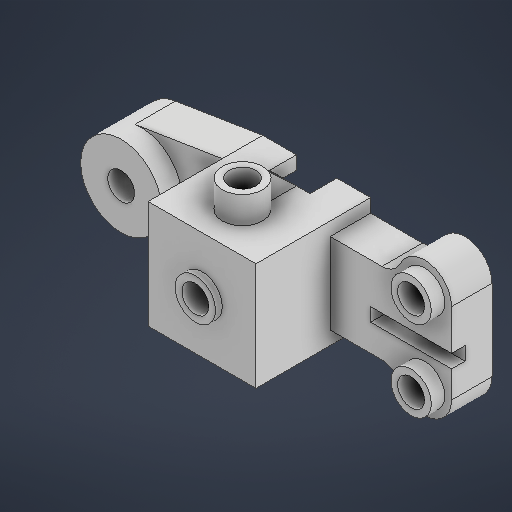
# Autodesk Inventor part: b5
Saved by Autodesk Inventor 2025.4 (Build 294407000, 407)
## iProperties
Created: 2026-05-15
Part Number: b5
Material: Generic
Document SubType Name: Modeling
Designer: VuQuan
Density: 1 g/cm^3
Appearance: Default
Author: VuQuan
Autodesk Inventor part; units mm, degrees
ref_plane "YZ Plane" through (0, 0, 0) normal (1, 0, 0) x (0, 1, 0)
ref_plane "XZ Plane" through (0, 0, 0) normal (0, 1, 0) x (-1, 0, 0)
ref_plane "XY Plane" through (0, 0, 0) normal (0, 0, 1) x (1, 0, 0)
sketch "Sketch1" plane through (0, 0, 0) normal (0, 0, 1) x (1, 0, 0)
  circle A0 centre (0, 0) radius 30
  line L0 (60, 40) -> (140, 40)
  line L1 (140, 40) -> (140, -40)
  line L2 (140, -40) -> (60, -40)
  line L3 (60, -40) -> (60, 40)
  line L4 (60, 40) -> (-4.7479, 29.6219)
  line L5 (60, -40) -> (-4.7479, -29.6219)
  line L6 (140, 30) -> (178.3772, 30)
  arc A1 (230, 30) -> (191.9298, 38.5714) centre (210, 30) ccw
  line L7 (230, 30) -> (230, -30)
  arc A2 (191.9298, -38.5714) -> (230, -30) centre (210, -30) ccw
  line L8 (178.3772, -30) -> (140, -30)
  arc A3 (178.3772, 30) -> (191.9298, 38.5714) centre (178.3772, 45) ccw
  arc A4 (191.9298, -38.5714) -> (178.3772, -30) centre (178.3772, -45) ccw
  point P0 (60, 0)
  point P1 (100, -40)
  point P2 (190, 30)
  point P3 (190, -30)
  point P4 (230, 0)
  point P5 (140, 0)
  dimension "d0" = 60
  dimension "d1" = 80
  dimension "d2" = 100
  dimension "d3" = 60
  dimension "d4" = 20
  dimension "d5" = 110
  dimension "d61" = 15
  constraints: 18 end point, 12 point on circle, 8 tangent, 7 point on line, 5 centre point, 4 midpoint, 4 perpendicular, 2 horizontal, 2 horizontal alignment, 2 parallel, 1 coincident, 1 equal radius, 1 vertical alignment
  measures "d0" diameter of A0
  measures "d1" distance of L1.end L2.end
  measures "d2" horizontal distance of point (100, -40) point (0, 0)
  measures "d3" distance between parallel lines of L8 L6
  measures "d4" radius of A1
  measures "d5" horizontal distance of A2.centre point (100, -40)
  measures "d61" radius of A3
extrude "Extrusion1" add sketch "Sketch1" along normal blind 45 contours A0
extrude "Extrusion2" add sketch "Sketch1" along normal blind 30 contours A0 L4 L3 L5 | L6 A3 A1 L7 A2 A4 L8 L1
extrude "Extrusion3" add sketch "Sketch1" along normal blind 85 contours L0 L1 L2 L3
hole "Hole1" at (0, 0, 0) direction (0, 0, 1) diameter 20 depth 45
sketch "Sketch2" plane through (0, 0, 0) normal (0, 0, -1) x (-1, 0, 0)
  circle A0 centre (0, 0) radius 10 projected
  line L0 (-60, 40) -> (4.7479, 29.6219) projected
  line L1 (4.7479, -29.6219) -> (-60, -40) projected
  line L2 (-50, 28.2695) -> (-50, -28.2695)
  line L3 (-50, -28.2695) -> (3.1653, -19.7479)
  arc A1 (3.1653, -19.7479) -> (3.1653, 19.7479) centre (0, 0) ccw
  line L4 (3.1653, 19.7479) -> (-50, 28.2695)
  line L5 (-60, 40) -> (-60, -40) projected
  dimension "d21" = 20
  dimension "d22" = 10
  constraints: 6 end point, 2 parallel, 2 point on circle, 2 tangent, 1 centre point, 1 coincident, 1 vertical
  measures "d21" radius of A1
  measures "d22" distance between parallel lines of L2 L5
extrude "Extrusion4" cut sketch "Sketch2" against normal blind 15
sketch "Sketch3" plane through (0, 0, 0) normal (0, 1, 0) x (-1, 0, 0)
  line L0 (-60, 85) -> (-25.09, 38.4533)
  line L1 (30, 45) -> (-30, 45) projected
  point P0 (0, 0)
  constraints: 2 end point, 1 point on line
extrude "Rib1" add sketch "Sketch3" along normal mid plane 10 rib yes fills toward (-42.585, 61.6966) open curves L0
sketch "Sketch4" plane through (0, 0, 0) normal (0, 0, -1) x (-1, 0, 0)
  line L0 (-140, 40) -> (-60, 40) projected
  line L1 (-140, -40) -> (-140, 40) projected
  line L2 (-140, -40) -> (-140, 40) projected
  line L3 (-140, 40) -> (-60, 40) projected
  line L4 (-60, 40) -> (-60, 5) projected
  line L5 (-60, 5) -> (-60, -5) projected
  line L6 (-60, -5) -> (-60, -40) projected
  line L7 (-60, -40) -> (-140, -40) projected
  line L8 (-70, 20) -> (-70, -20)
  arc A0 (-80, -30) -> (-70, -20) centre (-80, -20) ccw
  line L9 (-80, -30) -> (-120, -30)
  arc A1 (-130, -20) -> (-120, -30) centre (-120, -20) ccw
  line L10 (-130, -20) -> (-130, 20)
  arc A2 (-120, 30) -> (-130, 20) centre (-120, 20) ccw
  line L11 (-120, 30) -> (-80, 30)
  arc A3 (-70, 20) -> (-80, 30) centre (-80, 20) ccw
  dimension "d31" = 10
  dimension "d32" = 10
  dimension "d34" = 10
  dimension "d35" = 10
  constraints: 8 end point, 8 point on circle, 8 tangent, 4 centre point, 3 equal radius, 2 perpendicular, 2 vertical, 1 parallel
  measures "d31" radius of A2
  measures "d32" distance between parallel lines of L7 L9
  measures "d34" distance between parallel lines of L2 L10
  measures "d35" distance between parallel lines of L0 L11
extrude "Extrusion5" cut sketch "Sketch4" against normal blind 70 contours L8 A0 L9 A1 L10 A2 L11 A3
sketch "Sketch5" plane through (60, 40, 0) normal (0, 1, 0) x (1, 0, 0)
  line L0 (80, 0) -> (0, 0) projected
  line L1 (80, -85) -> (0, -85) projected
  circle A0 centre (40, -55) radius 10
  circle A1 centre (40, -55) radius 15
  point P0 (-60, 0)
  point P1 (40, -85)
  dimension "d38" = 20
  dimension "d39" = 30
  dimension "d40" = 55
  constraints: 2 centre point, 1 coincident, 1 midpoint, 1 vertical alignment
  measures "d38" diameter of A0
  measures "d39" diameter of A1
  measures "d40" distance from line of L0 A0.centre
extrude "Extrusion6" add sketch "Sketch5" along normal blind 20
extrude "Extrusion7" cut sketch "Sketch5" against normal up to surface (10 mm away) contours A0
sketch "Sketch6" plane through (60, 40, 0) normal (0, 1, 0) x (1, 0, 0)
  line L0 (80, 0) -> (0, 0) projected
  line L1 (55, 0) -> (55, -20)
  line L2 (55, -20) -> (25, -20)
  line L3 (25, -20) -> (25, 0)
  point P0 (-60, 0)
  point P1 (40, -20)
  point P2 (40, 0)
  dimension "d45" = 20
  dimension "d46" = 30
  constraints: 6 end point, 2 midpoint, 2 perpendicular, 2 point on line, 1 vertical, 1 vertical alignment
  measures "d45" distance of L1.start L1.end
  measures "d46" distance of L1.end L2.end
extrude "Extrusion8" cut sketch "Sketch6" against normal up to surface (80 mm away)
ref_plane "Work Plane1" through (100, 40, 0) normal (-1, 0, 0) x (0, 0, 1)
sketch "Sketch7" plane through (100, 40, 0) normal (-1, 0, 0) x (0, 0, 1)
  line L0 (20, 0) -> (41.4341, 20)
  line L1 (70, 20) -> (40, 20) projected
  point P0 (0, -40)
  constraints: 2 end point, 1 coincident, 1 point on line
extrude "Rib2" add sketch "Sketch7" along normal mid plane 10 rib yes fills toward (30.7511, 9.9634) open curves L0
sketch "Sketch8" plane through (0, 0, 85) normal (0, 0, 1) x (1, 0, 0)
  line L0 (140, 40) -> (60, 40) projected
  line L1 (140, -40) -> (140, 40) projected
  circle A0 centre (100, 0) radius 10
  circle A1 centre (100, 0) radius 15
  point P0 (0, 0)
  point P1 (140, 0)
  point P2 (100, 40)
  dimension "d55" = 20
  dimension "d56" = 30
  constraints: 2 centre point, 2 midpoint, 1 coincident, 1 horizontal alignment, 1 vertical alignment
  measures "d55" diameter of A0
  measures "d56" diameter of A1
extrude "Extrusion9" add sketch "Sketch8" along normal blind 5
extrude "Extrusion10" cut sketch "Sketch8" against normal up to surface (15 mm away) contours A0
sketch "Sketch9" plane through (230, -30, 0) normal (1, 0, 0) x (0, 0, -1)
  line L0 (-30, 0) -> (-30, 60) projected
  line L1 (-30, 30) -> (-20, 30)
  line L2 (-20, 30) -> (-20, 20)
  line L3 (-20, 20) -> (-30, 20)
  point P0 (0, 30)
  point P1 (-20, 25)
  point P2 (-30, 25)
  dimension "d62" = 10
  dimension "d63" = 10
  constraints: 6 end point, 2 midpoint, 2 perpendicular, 1 horizontal, 1 horizontal alignment, 1 point on line
  measures "d62" distance of L1.start L1.end
  measures "d63" distance of L1.end L2.end
extrude "Extrusion11" cut sketch "Sketch9" against normal blind 60
sketch "Sketch10" plane through (0, 0, 30) normal (0, 0, 1) x (1, 0, 0)
  arc A0 (230, 30) -> (191.9298, 38.5714) centre (210, 30) ccw projected
  arc A1 (191.9298, -38.5714) -> (230, -30) centre (210, -30) ccw projected
  circle A2 centre (210, -30) radius 15
  circle A3 centre (210, 30) radius 15
  circle A4 centre (210, -30) radius 10
  circle A5 centre (210, 30) radius 10
  circle A6 centre (210, 30) radius 5
  circle A7 centre (210, -30) radius 5
  point P0 (0, 0)
  dimension "d66" = 30
  dimension "d67" = 20
  dimension "d72" = 10
  constraints: 6 centre point, 6 coincident, 3 equal radius
  measures "d66" diameter of A2
  measures "d67" diameter of A4
  measures "d72" diameter of A6
extrude "Extrusion12" add sketch "Sketch10" along normal blind 10 contours A2 | A3
extrude "Extrusion13" cut sketch "Sketch10" against normal blind 5 contours A4 | A5 | A6 | A7
extrude "Extrusion14" cut sketch "Sketch10" against normal up to surface (30 mm away) contours A6 | A7
body "Solid1"
